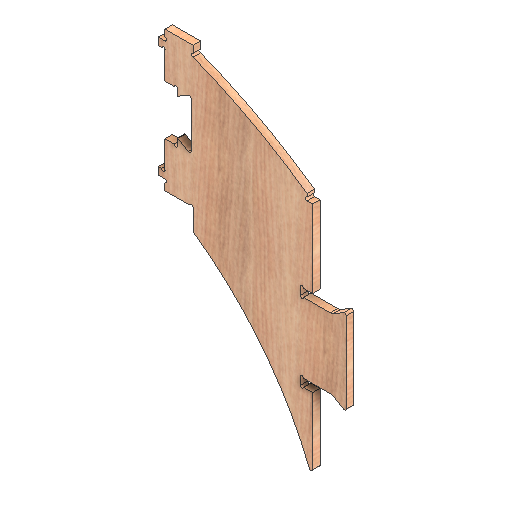
# Autodesk Inventor part: Support E
Saved by Autodesk Inventor 2021 (Build 250183000, 183)
## iProperties
Created: 2020-05-09
Part Number: Support E
Material: Wood (Birch)
Document SubType Name: Modeling
Designer: Dan Wikman
Density: 0.55 g/cm^3
Appearance: Birch - Natural Polished
Mass: 1550.62 g
Surface Area: 3587 cm^2
Volume: 2819.31 cm^3
Autodesk Inventor part; units mm, degrees
ref_plane "YZ Plane" through (0, 0, 0) normal (1, 0, 0) x (0, 1, 0)
ref_plane "XZ Plane" through (0, 0, 0) normal (0, 1, 0) x (-1, 0, 0)
ref_plane "XY Plane" through (0, 0, 0) normal (0, 0, 1) x (1, 0, 0)
sketch "CONTOURS" plane through (0, 0, 0) normal (0, 0, 1) x (1, 0, 0)
  arc A0 (2046.6196, 767.5507) -> (2038.9046, 766.0679) centre (2042.9046, 766.0679) ccw
  arc A1 (1973.7702, 871.0874) -> (1973.7702, 879.0874) centre (1973.7702, 875.0874) ccw
  line L0 (1957.6292, 879.0874) -> (1973.7702, 879.0874)
  line L1 (1957.6292, 897.0874) -> (1957.6292, 879.0874)
  line L2 (1965.7702, 897.0874) -> (1957.6292, 897.0874)
  arc A2 (1965.7702, 897.0874) -> (1973.7702, 897.0874) centre (1969.7702, 897.0874) ccw
  line L3 (1973.7702, 963.0802) -> (1973.7702, 897.0874)
  line L4 (1995.7702, 963.0802) -> (1973.7702, 963.0802)
  arc A3 (1995.7702, 963.0802) -> (2003.7702, 963.0802) centre (1999.7702, 963.0802) ccw
  line L5 (2003.7702, 979.652) -> (2003.7702, 963.0802)
  line L6 (2004.1939, 979.4354) -> (2003.7702, 979.652)
  line L7 (2004.6099, 979.2045) -> (2004.1939, 979.4354)
  line L8 (2029.7702, 964.6782) -> (2004.6099, 979.2045)
  arc A4 (2029.7702, 964.6782) -> (2037.2702, 969.0084) centre (2032.2702, 969.0084) ccw
  line L9 (2037.2702, 1077.5665) -> (2037.2702, 969.0084)
  arc A5 (2037.2702, 1077.5665) -> (2029.7702, 1081.8966) centre (2032.2702, 1077.5665) ccw
  line L10 (2004.6099, 1067.3703) -> (2029.7702, 1081.8966)
  line L11 (2004.1939, 1067.1394) -> (2004.6099, 1067.3703)
  arc A6 (2411.2702, 811.8331) -> (2405.2702, 815.2972) centre (2407.2702, 811.8331) ccw
  line L12 (2003.7702, 1066.9228) -> (2004.1939, 1067.1394)
  line L13 (2003.7702, 1083.4946) -> (2003.7702, 1066.9228)
  arc A7 (2003.7702, 1083.4946) -> (1995.7702, 1083.4947) centre (1999.7702, 1083.4947) ccw
  line L14 (1973.7702, 1083.4947) -> (1995.7702, 1083.4947)
  line L15 (1973.7702, 1149.4874) -> (1973.7702, 1083.4947)
  arc A8 (1973.7702, 1149.4874) -> (1965.7702, 1149.4874) centre (1969.7702, 1149.4874) ccw
  line L16 (1957.6292, 1149.4874) -> (1965.7702, 1149.4874)
  line L17 (1957.6292, 1167.4874) -> (1957.6292, 1149.4874)
  line L18 (1973.7702, 1167.4874) -> (1957.6292, 1167.4874)
  arc A9 (1973.7702, 1167.4874) -> (1973.7702, 1175.4874) centre (1973.7702, 1171.4874) ccw
  line L19 (1973.7702, 1192.2873) -> (1973.7702, 1175.4874)
  line L20 (2041.6292, 1192.2873) -> (1973.7702, 1192.2873)
  line L21 (2041.6292, 1175.5988) -> (2041.6292, 1192.2873)
  arc A10 (2041.6292, 1175.5988) -> (2041.6292, 1167.5988) centre (2041.6292, 1171.5988) ccw
  arc A11 (2316.6292, 1020.2242) -> (2041.6292, 1167.5988) centre (1569.4645, -43.7184) ccw
  line L22 (2316.6292, 1012.7612) -> (2316.6292, 1020.2242)
  arc A12 (2316.6292, 1012.7612) -> (2316.6292, 1004.7612) centre (2316.6292, 1008.7612) ccw
  line L23 (2330.1292, 1004.7612) -> (2316.6292, 1004.7612)
  line L24 (2330.1292, 817.7613) -> (2330.1292, 1004.7612)
  line L25 (2308.1292, 817.7613) -> (2330.1292, 817.7613)
  arc A13 (2308.1292, 817.7613) -> (2300.1292, 817.7613) centre (2304.1292, 817.7613) ccw
  line L26 (2300.1292, 798.7613) -> (2300.1292, 817.7613)
  arc A14 (2300.1292, 798.7613) -> (2308.1292, 798.7613) centre (2304.1292, 798.7613) ccw
  line L27 (2331.6292, 798.7613) -> (2308.1292, 798.7613)
  line L28 (2372.6099, 798.7613) -> (2331.6292, 798.7613)
  arc A15 (2372.6099, 798.7613) -> (2380.1099, 800.7709) centre (2372.6099, 813.7613) ccw
  line L29 (2405.2702, 815.2972) -> (2380.1099, 800.7709)
  line L30 (2411.2702, 616.6895) -> (2411.2702, 811.8331)
  arc A16 (2405.2702, 613.2254) -> (2411.2702, 616.6895) centre (2407.2702, 616.6895) ccw
  line L31 (2380.1099, 627.7517) -> (2405.2702, 613.2254)
  arc A17 (2380.1099, 627.7517) -> (2372.6099, 629.7613) centre (2372.6099, 614.7613) ccw
  line L32 (2331.6292, 629.7613) -> (2372.6099, 629.7613)
  line L33 (2308.1292, 629.7613) -> (2331.6292, 629.7613)
  arc A18 (2308.1292, 629.7613) -> (2300.1292, 629.7613) centre (2304.1292, 629.7613) ccw
  line L34 (2300.1292, 610.7613) -> (2300.1292, 629.7613)
  arc A19 (2300.1292, 610.7613) -> (2308.1292, 610.7613) centre (2304.1292, 610.7613) ccw
  line L35 (2330.1292, 610.7613) -> (2308.1292, 610.7613)
  line L36 (2330.1287, 449.505) -> (2330.1292, 610.7613)
  arc A20 (2322.4137, 448.0223) -> (2330.1287, 449.505) centre (2326.1287, 449.505) ccw
  arc A21 (2322.4137, 448.0223) -> (2041.6292, 802.4876) centre (1588.4809, 155.0905) ccw
  line L37 (2041.6292, 854.2873) -> (2041.6292, 802.4876)
  arc A22 (2041.6292, 854.2873) -> (2033.6292, 854.2873) centre (2037.6292, 854.2873) ccw
  line L38 (1973.7702, 854.2874) -> (2033.6292, 854.2873)
  line L39 (1973.7702, 871.0874) -> (1973.7702, 854.2874)
  constraints: 80 end point, 46 point on circle, 23 centre point
sketch "LETTERS" plane through (0, 0, 0) normal (0, 0, 1) x (1, 0, 0)
  line L0 (2195.1138, 872.4502) -> (2195.1138, 887.1377)
  line L1 (2195.1138, 887.1377) -> (2175.306, 887.1377)
  line L2 (2175.306, 887.1377) -> (2175.306, 872.4502)
  line L3 (2185.4137, 887.1672) -> (2185.4137, 876.5)
  constraints: 8 end point
extrude "Extrusion1" add sketch "CONTOURS" along normal blind 18
body "Solid1"
